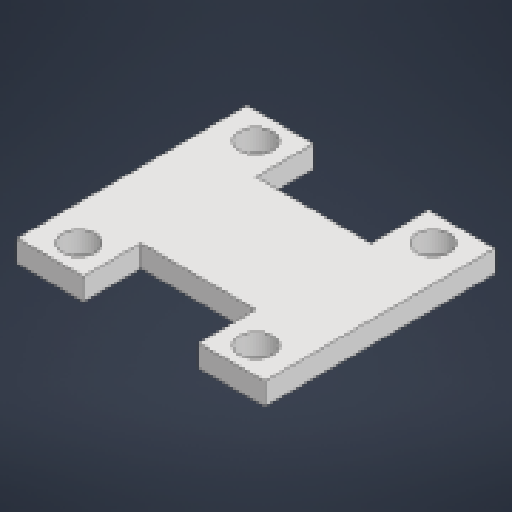
# Autodesk Inventor part: PCB_Housing_08_V4
Saved by Autodesk Inventor 2026.2 (Build 302298000, 298)
## iProperties
Created: 2026-03-23
Part Number: PCB_Housing_08_V4
Material: Generic
Document SubType Name: Modeling
Designer: vckot
Density: 1 g/cm^3
Appearance: Default
Author: vckot
Autodesk Inventor part; units mm, degrees
ref_plane "YZ Plane" through (0, 0, 0) normal (1, 0, 0) x (0, 1, 0)
ref_plane "XZ Plane" through (0, 0, 0) normal (0, 1, 0) x (-1, 0, 0)
ref_plane "XY Plane" through (0, 0, 0) normal (0, 0, 1) x (1, 0, 0)
sketch "Sketch1" plane through (0, 0, 0) normal (0, 1, 0) x (-1, 0, 0)
  line L0 (-6.5, 6.5) -> (6.5, 6.5)
  line L1 (6.5, 6.5) -> (6.5, -6.5)
  line L2 (6.5, -6.5) -> (-6.5, -6.5)
  line L3 (-6.5, -6.5) -> (-6.5, 6.5)
  line L4 (-6.5, 6.5) -> (6.5, -6.5) construction
  line L5 (6.5, 6.5) -> (-6.5, -6.5) construction
  circle A0 centre (10, 10) radius 2.375
  circle A1 centre (10, -10) radius 2.375
  circle A2 centre (-10, 10) radius 2.375
  circle A3 centre (-10, -10) radius 2.375
  line L6 (-14, 13) -> (14, 13)
  line L7 (14, 13) -> (14, -13)
  line L8 (14, -13) -> (-14, -13)
  line L9 (-14, -13) -> (-14, 13)
  line L10 (-14, 13) -> (14, -13) construction
  line L11 (14, 13) -> (-14, -13) construction
  line L12 (6.5, 6.5) -> (6.5, 13)
  line L13 (-6.5, 6.5) -> (-6.5, 13)
  line L14 (-6.5, -6.5) -> (-6.5, -13)
  line L15 (6.5, -6.5) -> (6.5, -13)
  point P0 (0, 0)
  dimension "d0" = 13
  dimension "d1" = 13
  dimension "d2" = 4.75
  dimension "d3" = 3.5
  dimension "d4" = 3.5
  dimension "d5" = 3.5
  dimension "d6" = 3.5
  dimension "d9" = 28
  dimension "d10" = 26
  constraints: 32 end point, 6 point on line, 4 centre point, 4 midpoint, 4 parallel, 3 equal radius, 3 perpendicular, 2 horizontal, 2 horizontal alignment, 2 vertical alignment, 1 vertical
  measures "d0" distance of L1.end L2.end
  measures "d1" distance of L0.end L1.end
  measures "d2" diameter of A0
  measures "d3" distance from line of L1 A1.centre
  measures "d4" distance from line of L2 A1.centre
  measures "d5" distance from line of L3 A3.centre
  measures "d6" distance from line of A2.centre L0
  measures "d9" distance between parallel lines of L9 L7
  measures "d10" distance between parallel lines of L6 L8
extrude "Extrusion1" add sketch "Sketch1" along normal blind 5 contours L3 L14 L8 L9 L6 L13 | L12 L6 L7 L8 L15 L1
extrude "Extrusion2" add sketch "Sketch1" along normal blind 2.5 contours L0 L1 L2 L3
body "Solid1"
